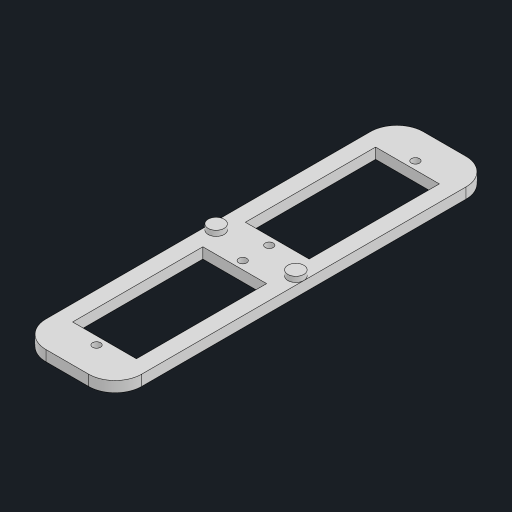
# Autodesk Inventor part: ServoMotor_Holder_V2
Saved by Autodesk Inventor 2023 (Build 270158000, 158)
## iProperties
Created: 2022-07-14
Part Number: ServoMotor_Holder_V2
Material: 一般
Document SubType Name: Modeling
Designer: legot
Density: 1 g/cm^3
Appearance: 既定
Author: legot
Autodesk Inventor part; units mm, degrees
ref_plane "YZ Plane" through (0, 0, 0) normal (1, 0, 0) x (0, 1, 0)
ref_plane "XZ Plane" through (0, 0, 0) normal (0, 1, 0) x (-1, 0, 0)
sketch "スケッチ1" plane through (0, 0, 0) normal (0, 1, 0) x (-1, 0, 0)
  line L0 (6, 12.25) -> (-6, 12.25)
  line L1 (-6, 12.25) -> (-6, -12.25)
  line L2 (-6, -12.25) -> (6, -12.25)
  line L3 (6, -12.25) -> (6, 12.25)
  line L4 (9, 19.25) -> (-9, 19.25)
  line L5 (-9, 19.25) -> (-9, -16.25)
  line L6 (-9, -16.25) -> (9, -16.25)
  line L7 (9, -16.25) -> (9, 19.25)
  line L8 (0, -13.75) -> (0, 13.75) construction
  point P0 (0, 0)
  point P1 (6, 0)
  point P2 (0, 12.25)
  point P3 (0, 19.25)
  point P4 (9, 1.5)
  point P5 (0, 0)
  dimension "d0" = 24.5
  dimension "d1" = 12
  dimension "d2" = 3
  dimension "d3" = 4
  dimension "d4" = 7
  dimension "d8" = 27.5
  constraints: 18 end point, 5 midpoint, 4 parallel, 2 horizontal, 2 perpendicular, 2 vertical alignment, 1 coincident, 1 horizontal alignment, 1 vertical
  measures "d0" distance of L2.end L0.start
  measures "d1" distance of L0.start L0.end
  measures "d2" distance between parallel lines of L7 L3
  measures "d3" distance between parallel lines of L6 L2
  measures "d4" distance between parallel lines of L0 L4
  measures "d8" distance of L8.start L8.end
extrude "押し出し1" add sketch "スケッチ1" along normal blind 2
hole "穴1" at (0, 0, -13.75) at (0, 0, 13.75) direction (0, 1, 0) diameter 1.5 end through all
mirror "ミラー1" about plane through (9, 0, -16.25) normal (0, 0, -1) of "押し出し1", "穴1"
fillet "フィレット1" radius 5 4 edges at (-9, 1, 19.25) (9, 1, 19.25) (9, 1, -51.75) (-9, 1, -51.75)
ref_plane "位置合わせ" through (-6, 0, -16.25) normal (0, 0, 1) x (1, 0, 0)
sketch "スケッチ2" plane through (0, 2, 0) normal (0, 1, 0) x (1, 0, 0)
  line L0 (-9, -14.25) -> (-9, 46.75) projected
  line L1 (9, -14.25) -> (9, 46.75) projected
  circle A0 centre (0, 18.75) radius 0.75 projected
  circle A1 centre (0, 13.75) radius 0.75 projected
  circle A2 centre (7.5, 16.25) radius 1.5
  circle A3 centre (-7.5, 16.25) radius 1.5
  line L2 (0, 18.75) -> (0, 13.75) construction
  point P0 (0, 0)
  point P1 (0, 16.25)
  dimension "d16" = 3
  constraints: 2 centre point, 2 end point, 2 horizontal alignment, 2 tangent, 1 equal radius, 1 midpoint, 1 vertical
  measures "d16" diameter of A2
extrude "押し出し2" add sketch "スケッチ2" along normal blind 1 contours A2 | A3
